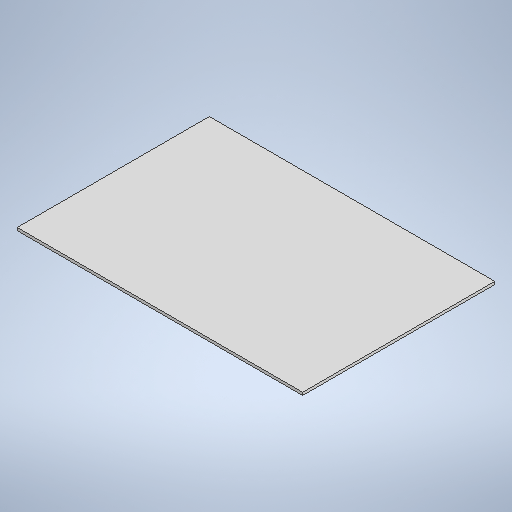
# Autodesk Inventor part: BSH 038 divider
Saved by Autodesk Inventor 2025 (Build 290162010, 162A)
## iProperties
Created: 2024-07-23
Part Number: BSH 038 divider
Material: Water
Document SubType Name: Sheet Metal
Designer: admin
Mass: 193.748 g
Surface Area: 1324.97 cm^2
Volume: 194.078 cm^3
Density: 0.9983 g/cm^3
Sheet Metal Rule: AISI304 3mm Die 32
Sheet Metal Width: 208,686 mm
Sheet Metal Length: 310,000 mm
Sheet Metal Area: 64692,660 mm^2
Appearance: Default
Flat Pattern Width: 20.8686 cm
Flat Pattern Length: 31 cm
Flat Pattern Area: 646.927 cm^2
Author: admin
Autodesk Inventor part; units mm, degrees
ref_plane "YZ Plane" through (0, 0, 0) normal (1, 0, 0) x (0, 1, 0)
ref_plane "XZ Plane" through (0, 0, 0) normal (0, 1, 0) x (-1, 0, 0)
ref_plane "XY Plane" through (0, 0, 0) normal (0, 0, 1) x (1, 0, 0)
sketch "Sketch6" plane through (0, 0, 0) normal (0, 0, 1) x (1, 0, 0)
  line L0 (155, 104.343) -> (-155, 104.343)
  line L1 (-155, 104.343) -> (-155, -104.343)
  line L2 (-155, -104.343) -> (155, -104.343)
  line L3 (155, -104.343) -> (155, 104.343)
  line L4 (155, 104.343) -> (-155, -104.343) construction
  line L5 (-155, 104.343) -> (155, -104.343) construction
  point P0 (0, 0)
  dimension "d40" = 310
  dimension "d41" = 208.686
  measures "d40" distance of L2.end L1.end
  measures "d41" distance of L1.end L0.end
extrude "Plate5" add sketch "Sketch6" along normal blind 3
equation "\"d42\" = Thickness"
equation "\"BendReliefWidth\" = Thickness"
equation "\"BendReliefDepth\" = 0.5 * Thickness"
equation "\"CornerReliefSize\" = 4 * Thickness"
equation "\"MinimumRemnant\" = 2 * Thickness"
equation "\"TransitionRadius\" = BendRadius"
equation "\"JacobiRadiusSize\" = BendRadius"
equation "\"GapSize\" = Thickness"
equation "\"Thickness\" = 3"
equation "\"BendRadius\" = 5"
body "Solid4"
